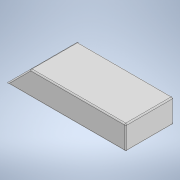
# Autodesk Inventor part: union_ruedas
Saved by Autodesk Inventor 2021 (Build 250183000, 183)
## iProperties
Created: 2022-01-26
Part Number: union_ruedas
Material: Genérico
Document SubType Name: Modeling
Designer: arthu
Density: 1 g/cm^3
Appearance: Valor por defecto
Author: arthu
Autodesk Inventor part; units mm, degrees
ref_plane "YZ Plane" through (0, 0, 0) normal (1, 0, 0) x (0, 1, 0)
ref_plane "XZ Plane" through (0, 0, 0) normal (0, 1, 0) x (-1, 0, 0)
ref_plane "XY Plane" through (0, 0, 0) normal (0, 0, 1) x (1, 0, 0)
sketch "Boceto1" plane through (0, 0, 0) normal (0, 0, 1) x (1, 0, 0)
  line L0 (100, -20) -> (-100, -20)
  line L1 (-60, 20) -> (100, 20)
  line L2 (100, 20) -> (100, -20)
  line L3 (100, -20) -> (-66.6667, 13.3333) construction
  line L4 (-100, -20) -> (100, 20) construction
  line L5 (-100, -20) -> (-60, 20)
  line L6 (-100, -20) -> (-43.4315, -20) construction
  point P0 (0, 0)
  dimension "d2" = 45
  constraints: 14 end point, 2 horizontal, 2 point on line, 1 equal length, 1 midpoint, 1 parallel
  measures "d2" angle of L6 L5
extrude "Extrusión1" add sketch "Boceto1" along normal blind 80
fillet "Empalme1" radius 2 11 edges at (20, 20, 0) (20, 20, 80) (0, -20, 0) (0, -20, 80) (-80, 0, 80) (-60, 20, 40) (-80, 0, 0) (100, 20, 40) (100, 0, 80) (100, 0, 0) (100, -20, 40)
